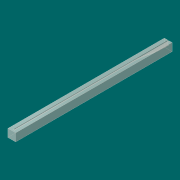
# Autodesk Inventor part: Scintillator Tile
Saved by Autodesk Inventor 2016 (Build 200138000, 138)
## iProperties
Created: 2015-08-14
Part Number: Scintillator Tile
Material: ABS Plastic
Document SubType Name: Modeling
Designer: Cosmic
Density: 1.06 g/cm^3
Appearance: Clear
Author: Cosmic
Autodesk Inventor part; units mm, degrees
ref_plane "YZ Plane" through (0, 0, 0) normal (1, 0, 0) x (0, 1, 0)
ref_plane "XZ Plane" through (0, 0, 0) normal (0, 1, 0) x (-1, 0, 0)
ref_plane "XY Plane" through (0, 0, 0) normal (0, 0, 1) x (1, 0, 0)
sketch "Sketch1" plane through (0, 0, 0) normal (0, 0, 1) x (1, 0, 0)
  line L0 (-5, -100) -> (5, -100)
  line L1 (5, -100) -> (5, 100)
  line L2 (5, 100) -> (-5, 100)
  line L3 (-5, 100) -> (-5, -100)
  line L4 (-5, -100) -> (5, 100) construction
  line L5 (5, -100) -> (-5, 100) construction
  point P0 (0, 0)
  dimension "d0" = 10
  dimension "d1" = 200
  constraints: 12 end point, 2 midpoint, 2 parallel, 1 horizontal, 1 perpendicular
  measures "d0" distance of L2.end L1.end
  measures "d1" distance of L1.end L0.end
extrude "Extrusion1" add sketch "Sketch1" along normal blind 10
sketch "Sketch12" plane through (5, -100, 0) normal (1, 0, 0) x (0, 0, -1)
  line L0 (0, 0) -> (0, 200) projected
  line L1 (0, 200) -> (-10, 200) projected
  line L2 (-10, 0) -> (-10, 200) projected
  line L3 (0, 0) -> (-10, 0) projected
  line L4 (-8.8, 0) -> (-8.8, 154.8445)
  arc A0 (-6.6, 174.6222) -> (-8.8, 154.8445) centre (81.2, 154.8445) ccw
  arc A1 (-6.6, 174.6222) -> (-4.4, 194.4) centre (-94.4, 194.4) ccw
  line L5 (-4.4, 194.4) -> (-4.4, 200)
  line L6 (0, 200) -> (-10, 200) projected
  line L7 (0, 0) -> (0, 200) projected
  point P0 (0, 100)
  dimension "d87" = 5.6
  dimension "d88" = 1.2
  dimension "d89" = 90
  dimension "d90" = 90
  dimension "d91" = 5.6
  constraints: 4 end point, 4 point on circle, 3 tangent, 2 centre point, 2 parallel, 2 point on line
  measures "d87" distance between parallel lines of L2 L5
  measures "d88" distance between parallel lines of L2 L4
  measures "d89" radius of A1
  measures "d90" radius of A0
  measures "d91" distance of L5.end L5.start
extrude "Extrusion13" cut sketch "Sketch12" against normal through all contours L3 L4 A0 A1 L5 L1 L0 keep common part
sketch "Sketch22" plane through (0, 0, 0) normal (0, 0, -1) x (-1, 0, 0)
  line L0 (5, -100) -> (-5, -100) projected
  line L1 (5, 100) -> (5, -100) projected
  line L2 (-5, 100) -> (5, 100) projected
  line L3 (-5, -100) -> (-5, 100) projected
  line L4 (5, -100) -> (-5, -100) projected
  line L5 (0.6, 100) -> (-0.6, 100)
  line L6 (-0.6, 100) -> (-0.6, -100)
  line L7 (-0.6, -100) -> (0.6, -100)
  line L8 (0.6, -100) -> (0.6, 100)
  line L9 (0.6, 100) -> (-0.6, -100) construction
  line L10 (-0.6, 100) -> (0.6, -100) construction
  point P0 (0, 0)
  dimension "d135" = 1.2
  constraints: 12 end point, 2 midpoint, 2 parallel, 1 horizontal, 1 perpendicular, 1 point on line
  measures "d135" distance between parallel lines of L6 L8
extrude "Extrusion22" add sketch "Sketch22" against normal blind 10 contours L0 L8 L2 L1 | L0 L3 L2 L6
sketch "Sketch23" plane through (-0.6, -100, 8.8) normal (0, 0, 1) x (1, 0, 0)
  line L0 (0, 154.8445) -> (0, 0) projected
  line L1 (0, 0) -> (1.2, 0) projected
  line L2 (1.2, 0) -> (1.2, 154.8445) projected
  line L3 (1.2, 154.8445) -> (0, 154.8445) projected
  line L4 (0, 0) -> (1.2, 0)
  line L5 (1.2, 0) -> (1.2, 3)
  line L6 (1.2, 3) -> (0, 3)
  line L7 (0, 3) -> (0, 0)
  point P0 (0.6, 100)
  dimension "d138" = 3
  constraints: 8 end point, 2 parallel, 1 horizontal, 1 perpendicular, 1 point on line
  measures "d138" distance between parallel lines of L1 L6
extrude "Extrusion23" add sketch "Sketch23" along normal up to surface (1.2 mm away) contours L6 L2 L1 L0
fillet "Fillet3" radius 0.6 8 edges at (-0.6, 84.4501, 4.9517) (-0.6, 64.7943, 8.2483) (-0.6, -21.0778, 8.8) (-0.6, 97.2, 4.4) (0.6, 84.4501, 4.9517) (0.6, 64.7943, 8.2483) (0.6, -21.0778, 8.8) (0.6, 97.2, 4.4)
equation "\"d0\" = ScintillatorWidth"
equation "\"d1\" = ScintillatorHeight"
equation "\"d2\" = ScintillatorThickness"
equation "\"d87\" = DeepTrackDepth"
equation "\"d88\" = ShallowTrackDepth"
equation "\"d89\" = LoopSmallTrackDiameter"
equation "\"d90\" = LoopSmallTrackDiameter"
equation "\"d91\" = DeepTrackDepth"
equation "\"d5\" = OpticalFiberDiameter + 2 * OpticalFiberClearence"
equation "\"d21\" = d5"
equation "\"d22\" = d5"
equation "\"OpticalFiberDiameter\" = 1"
equation "\"ScintillatorThickness\" = 10"
equation "\"OpticalFiberClearence\" = 0.1"
equation "\"SmallTrackDiameter\" = 175"
equation "\"ScintillatorEdgeClearence\" = 3"
equation "\"ScintillatorWidth\" = 10"
equation "\"ScintillatorHeight\" = 200"
equation "\"ShallowTrackDepth\" = 1.2"
equation "\"MPPCClearence\" = 0.075"
equation "\"MPPCSensorClearence\" = 1.45"
equation "\"MPPCSensorOffsett\" = 2.105"
equation "\"MPPCWidth\" = 5.9"
equation "\"MPPCHeight\" = 6.55"
equation "\"FiberEdgeOffsett\" = 5"
equation "\"MPPCDepth\" = 1"
equation "\"LongFiberAngle\" = 30deg"
equation "\"ShortFiberAngle\" = 78deg"
equation "\"LoopLargeTrackRatio\" = 1.1"
equation "\"LoopSmallTrackDiameter\" = 90"
equation "\"FiberSensorClerence\" = 0.5"
equation "\"MountingScrewOffsett\" = 9"
equation "\"MountingScrewDepth\" = 4"
equation "\"DeepTrackDepth\" = 5.6"
equation "\"FoilThickness\" = 0.2"
equation "\"silveringThickness\" = 0.2"
equation "\"rubberizedCoating\" = 0.5"
body "Solid1"
